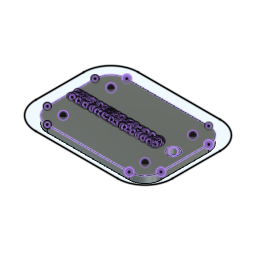
key chain mold v3 (Autodesk Fusion 360 design; units mm, degrees)
Autodesk Fusion 360 part; units mm, degrees
sketch "Sketch1" plane through (0, 0, 0) normal (0, 0, 1) x (1, 0, 0) in component "KEY CHAIN"
  line L0 (0, 0) -> (50, 0)
  line L1 (50, 0) -> (50, 35)
  line L2 (50, 35) -> (0, 35)
  line L3 (0, 35) -> (0, 0)
  dimension "d1" = 50
  dimension "d2" = 35
  constraint horizontal L0
  constraint vertical L1
  constraint horizontal L2
  constraint vertical L3
  constraint coincident L0.start L3.end
  measures "d1" distance of L0.start L0.end
  measures "d2" distance of L0.start L2.end
extrude "Extrude1" add sketch "Sketch1" along normal blind 3 in component "KEY CHAIN"
fillet "Fillet1" radius 7 4 edges at (0, 35, 1.5) (0, 0, 1.5) (50, 0, 1.5) (50, 35, 1.5) in component "KEY CHAIN"
sketch "Sketch2" plane through (0, 0, 3) normal (0, 0, 1) x (-1, 0, 0) in component "KEY CHAIN"
  arc A0 (-50, -28) -> (-43, -35) centre (-43, -28) ccw
  line L0 (-43, -35) -> (-7, -35)
  arc A1 (-7, -35) -> (0, -28) centre (-7, -28) ccw
  line L1 (0, -28) -> (0, -7)
  arc A2 (0, -7) -> (-7, 0) centre (-7, -7) ccw
  line L2 (-7, 0) -> (-43, 0)
  arc A3 (-43, 0) -> (-50, -7) centre (-43, -7) ccw
  line L3 (-50, -7) -> (-50, -28)
  line L4 (-50, -17.5) -> (-45, -17.5) construction
  dimension "d7" = 5
  constraint midpoint L3 L4.start
  constraint perpendicular L3 L4
  measures "d7" distance of L4.start L4.end
hole "Hole1" at (45, 17.5, 3) direction (0, 0, -1) diameter 5 depth 3 tip angle 180 in component "KEY CHAIN"
sketch "Sketch3" plane through (0, 0, 3) normal (0, 0, 1) x (-1, 0, 0) in component "KEY CHAIN"
  circle A0 centre (-45, -17.5) radius 2.5
  arc A1 (-50, -28) -> (-43, -35) centre (-43, -28) ccw
  line L0 (-43, -35) -> (-7, -35)
  arc A2 (-7, -35) -> (0, -28) centre (-7, -28) ccw
  line L1 (0, -28) -> (0, -7)
  arc A3 (0, -7) -> (-7, 0) centre (-7, -7) ccw
  line L2 (-7, 0) -> (-43, 0)
  arc A4 (-43, 0) -> (-50, -7) centre (-43, -7) ccw
  line L3 (-50, -7) -> (-50, -28)
  line L4 (0, 0) -> (-40, 0) construction
  line L5 (-40, 0) -> (-40, -35) construction
  line L6 (-40, -35) -> (0, -35) construction
  line L7 (0, -35) -> (0, 0) construction
  dimension "d11" = 3
  text T0 "PHILLYSNEXT LLC" font "Arial" height 3 bold align centre middle in box 40 x 35 at (0, 0) x (-1, 0) y (0, -1) spacing 1 kerned
  constraint coincident L2
extrude "Extrude2" add sketch "Sketch3" along normal blind 1 text T0 in component "KEY CHAIN"
sketch "Sketch1 (2)" plane through (0, 0, 3) normal (0, 0, 1) x (-1, 0, 0) in component "ONE PART MOLD"
  arc A0 (-50, -28) -> (-43, -35) centre (-43, -28) ccw
  line L0 (-43, -35) -> (-7, -35)
  arc A1 (-7, -35) -> (0, -28) centre (-7, -28) ccw
  line L1 (0, -28) -> (0, -7)
  arc A2 (0, -7) -> (-7, 0) centre (-7, -7) ccw
  line L2 (-7, 0) -> (-43, 0)
  arc A3 (-43, 0) -> (-50, -7) centre (-43, -7) ccw
  line L3 (-50, -7) -> (-50, -28)
  circle A4 centre (-45, -17.5) radius 2.5
  line L4 (-4.1569, -16) -> (-4.1569, -19)
  line L5 (-4.1569, -19) -> (-4.7626, -19)
  line L6 (-4.7626, -19) -> (-4.7626, -17.8192)
  line L7 (-4.7626, -17.8192) -> (-5.9495, -17.8192)
  line L8 (-5.9495, -17.8192) -> (-5.9495, -19)
  line L9 (-5.9495, -19) -> (-6.5553, -19)
  line L10 (-6.5553, -19) -> (-6.5553, -16)
  line L11 (-6.5553, -16) -> (-5.9495, -16)
  line L12 (-5.9495, -16) -> (-5.9495, -17.3117)
  line L13 (-5.9495, -17.3117) -> (-4.7626, -17.3117)
  line L14 (-4.7626, -17.3117) -> (-4.7626, -16)
  line L15 (-4.7626, -16) -> (-4.1569, -16)
  line L16 (-8.3622, -16) -> (-8.3622, -18.9754)
  line L17 (-8.3622, -18.9754) -> (-8.9679, -18.9754)
  line L18 (-8.9679, -18.9754) -> (-8.9679, -16.5055)
  line L19 (-8.9679, -16.5055) -> (-10.4741, -16.5055)
  line L20 (-10.4741, -16.5055) -> (-10.4741, -16)
  line L21 (-10.4741, -16) -> (-8.3622, -16)
  line L22 (-13.869, -16) -> (-13.869, -17.2626)
  line L23 (-13.869, -17.2626) -> (-12.7701, -19)
  line L24 (-12.7701, -19) -> (-13.4802, -19)
  line L25 (-13.4802, -19) -> (-14.1862, -17.8131)
  line L26 (-14.1862, -17.8131) -> (-14.8779, -19)
  line L27 (-14.8779, -19) -> (-15.5757, -19)
  line L28 (-15.5757, -19) -> (-14.4727, -17.2585)
  line L29 (-14.4727, -17.2585) -> (-14.4727, -16)
  line L30 (-14.4727, -16) -> (-13.869, -16)
  line L31 (-38.0532, -17.103) -> (-38.6405, -16.9168)
  spline S0 degree 3 poles (-38.6405, -16.9168) (-38.5921, -16.7668) (-38.5015, -16.4863) (-38.2899, -16.2822) (-38.1913, -16.1872) knots 0 0 0 0 0.04642 0.086856 0.086856 0.086856 0.086856
  spline S1 degree 3 poles (-38.1913, -16.1872) (-38.0756, -16.1178) (-37.8308, -15.9708) (-37.545, -15.9564) (-37.3943, -15.9488) knots 0 0 0 0 0.039867 0.084342 0.084342 0.084342 0.084342
  spline S2 degree 3 poles (-37.3943, -15.9488) (-37.2051, -15.9646) (-36.8336, -15.9956) (-36.5508, -16.238) (-36.412, -16.3571) knots 0 0 0 0 0.055382 0.108818 0.108818 0.108818 0.108818
  spline S3 degree 3 poles (-36.412, -16.3571) (-36.2999, -16.5125) (-36.0603, -16.8446) (-36.0388, -17.255) (-36.0273, -17.4734) knots 0 0 0 0 0.056279 0.120316 0.120316 0.120316 0.120316
  spline S4 degree 3 poles (-36.0273, -17.4734) (-36.0378, -17.7027) (-36.0574, -18.1287) (-36.3014, -18.4763) (-36.4141, -18.6368) knots 0 0 0 0 0.067232 0.124868 0.124868 0.124868 0.124868
  spline S5 degree 3 poles (-36.4141, -18.6368) (-36.5561, -18.7576) (-36.849, -19.0068) (-37.2332, -19.0361) (-37.4311, -19.0512) knots 0 0 0 0 0.054496 0.112371 0.112371 0.112371 0.112371
  spline S6 degree 3 poles (-37.4311, -19.0512) (-37.6033, -19.04) (-37.9339, -19.0187) (-38.1986, -18.8206) (-38.3254, -18.7258) knots 0 0 0 0 0.05054 0.097009 0.097009 0.097009 0.097009
  spline S7 degree 3 poles (-38.3254, -18.7258) (-38.3904, -18.6507) (-38.531, -18.4883) (-38.5969, -18.2834) (-38.6323, -18.1733) knots 0 0 0 0 0.02949 0.063785 0.063785 0.063785 0.063785
  line L32 (-38.6323, -18.1733) -> (-38.0327, -18.03)
  spline S8 degree 3 poles (-38.0327, -18.03) (-38.011, -18.103) (-37.9687, -18.2451) (-37.8624, -18.3482) (-37.8107, -18.3984) knots 0 0 0 0 0.02243 0.043656 0.043656 0.043656 0.043656
  spline S9 degree 3 poles (-37.8107, -18.3984) (-37.7503, -18.4377) (-37.6256, -18.519) (-37.477, -18.5285) (-37.4004, -18.5334) knots 0 0 0 0 0.021266 0.043851 0.043851 0.043851 0.043851
  spline S10 degree 3 poles (-37.4004, -18.5334) (-37.295, -18.524) (-37.0872, -18.5056) (-36.9344, -18.3638) (-36.8591, -18.294) knots 0 0 0 0 0.030797 0.060705 0.060705 0.060705 0.060705
  spline S11 degree 3 poles (-36.8591, -18.294) (-36.7989, -18.1919) (-36.6586, -17.9543) (-36.654, -17.6767) (-36.6514, -17.5184) knots 0 0 0 0 0.035017 0.081505 0.081505 0.081505 0.081505
  spline S12 degree 3 poles (-36.6514, -17.5184) (-36.6532, -17.3518) (-36.6562, -17.0633) (-36.7967, -16.8135) (-36.8561, -16.708) knots 0 0 0 0 0.048972 0.084763 0.084763 0.084763 0.084763
  spline S13 degree 3 poles (-36.8561, -16.708) (-36.9299, -16.6376) (-37.0791, -16.4954) (-37.2844, -16.4762) (-37.3881, -16.4666) knots 0 0 0 0 0.029695 0.059976 0.059976 0.059976 0.059976
  spline S14 degree 3 poles (-37.3881, -16.4666) (-37.4655, -16.4727) (-37.6185, -16.4848) (-37.7423, -16.5753) (-37.8035, -16.6201) knots 0 0 0 0 0.022784 0.04507 0.04507 0.04507 0.04507
  spline S15 degree 3 poles (-37.8035, -16.6201) (-37.8584, -16.6832) (-37.9803, -16.8234) (-38.0273, -17.0038) (-38.0532, -17.103) knots 0 0 0 0 0.024761 0.055018 0.055018 0.055018 0.055018
  line L33 (-21.6985, -16) -> (-21.6985, -19)
  line L34 (-21.6985, -19) -> (-23.9229, -19)
  line L35 (-23.9229, -19) -> (-23.9229, -18.4925)
  line L36 (-23.9229, -18.4925) -> (-22.3042, -18.4925)
  line L37 (-22.3042, -18.4925) -> (-22.3042, -17.8274)
  line L38 (-22.3042, -17.8274) -> (-23.8104, -17.8274)
  line L39 (-23.8104, -17.8274) -> (-23.8104, -17.322)
  line L40 (-23.8104, -17.322) -> (-22.3042, -17.322)
  line L41 (-22.3042, -17.322) -> (-22.3042, -16.5055)
  line L42 (-22.3042, -16.5055) -> (-23.9802, -16.5055)
  line L43 (-23.9802, -16.5055) -> (-23.9802, -16)
  line L44 (-23.9802, -16) -> (-21.6985, -16)
  line L45 (-27.9645, -16) -> (-27.9645, -18.4925)
  line L46 (-27.9645, -18.4925) -> (-27.0744, -18.4925)
  line L47 (-27.0744, -18.4925) -> (-27.0744, -19)
  line L48 (-27.0744, -19) -> (-29.4584, -19)
  line L49 (-29.4584, -19) -> (-29.4584, -18.4925)
  line L50 (-29.4584, -18.4925) -> (-28.5703, -18.4925)
  line L51 (-28.5703, -18.4925) -> (-28.5703, -16)
  line L52 (-28.5703, -16) -> (-27.9645, -16)
  line L53 (-33.59, -16) -> (-33.59, -18.9754)
  line L54 (-33.59, -18.9754) -> (-34.1958, -18.9754)
  line L55 (-34.1958, -18.9754) -> (-34.1958, -16.5055)
  line L56 (-34.1958, -16.5055) -> (-35.7019, -16.5055)
  line L57 (-35.7019, -16.5055) -> (-35.7019, -16)
  line L58 (-35.7019, -16) -> (-33.59, -16)
  line L59 (-31.03, -16) -> (-31.03, -18.9754)
  line L60 (-31.03, -18.9754) -> (-31.6357, -18.9754)
  line L61 (-31.6357, -18.9754) -> (-31.6357, -16.5055)
  line L62 (-31.6357, -16.5055) -> (-33.1419, -16.5055)
  line L63 (-33.1419, -16.5055) -> (-33.1419, -16)
  line L64 (-33.1419, -16) -> (-31.03, -16)
  line L65 (-24.1889, -16) -> (-25.2142, -17.5655)
  line L66 (-25.2142, -17.5655) -> (-24.2851, -19)
  line L67 (-24.2851, -19) -> (-24.9932, -19)
  line L68 (-24.9932, -19) -> (-25.5948, -18.0362)
  line L69 (-25.5948, -18.0362) -> (-26.1842, -19)
  line L70 (-26.1842, -19) -> (-26.8861, -19)
  line L71 (-26.8861, -19) -> (-25.9529, -17.543)
  line L72 (-25.9529, -17.543) -> (-26.9782, -16)
  line L73 (-26.9782, -16) -> (-26.2476, -16)
  line L74 (-26.2476, -16) -> (-25.5825, -17.0375)
  line L75 (-25.5825, -17.0375) -> (-24.9154, -16)
  line L76 (-24.9154, -16) -> (-24.1889, -16)
  line L77 (-18.678, -16) -> (-18.678, -19)
  line L78 (-18.678, -19) -> (-19.2674, -19)
  line L79 (-19.2674, -19) -> (-20.4952, -16.9966)
  line L80 (-20.4952, -16.9966) -> (-20.4952, -19)
  line L81 (-20.4952, -19) -> (-21.058, -19)
  line L82 (-21.058, -19) -> (-21.058, -16)
  line L83 (-21.058, -16) -> (-20.4502, -16)
  line L84 (-20.4502, -16) -> (-19.2408, -17.9563)
  line L85 (-19.2408, -17.9563) -> (-19.2408, -16)
  line L86 (-19.2408, -16) -> (-18.678, -16)
  line L87 (-15.7231, -16.9761) -> (-16.3124, -17.0334)
  spline S16 degree 3 poles (-16.3124, -17.0334) (-16.3318, -16.9438) (-16.3672, -16.7797) (-16.478, -16.6544) (-16.5283, -16.5975) knots 0 0 0 0 0.026965 0.049368 0.049368 0.049368 0.049368
  spline S17 degree 3 poles (-16.5283, -16.5975) (-16.5901, -16.557) (-16.7229, -16.4699) (-16.8821, -16.4624) (-16.9673, -16.4584) knots 0 0 0 0 0.021772 0.046802 0.046802 0.046802 0.046802
  spline S18 degree 3 poles (-16.9673, -16.4584) (-17.0552, -16.4608) (-17.2133, -16.4652) (-17.3483, -16.5462) (-17.4083, -16.5822) knots 0 0 0 0 0.025843 0.046491 0.046491 0.046491 0.046491
  spline S19 degree 3 poles (-17.4083, -16.5822) (-17.4515, -16.6239) (-17.5343, -16.7037) (-17.5494, -16.8174) (-17.5566, -16.8718) knots 0 0 0 0 0.01744 0.033404 0.033404 0.033404 0.033404
  spline S20 degree 3 poles (-17.5566, -16.8718) (-17.5543, -16.9056) (-17.5497, -16.9716) (-17.5124, -17.0262) (-17.4942, -17.0529) knots 0 0 0 0 0.009971 0.019467 0.019467 0.019467 0.019467
  spline S21 degree 3 poles (-17.4942, -17.0529) (-17.4667, -17.0779) (-17.4031, -17.1358) (-17.3222, -17.1658) (-17.2763, -17.1828) knots 0 0 0 0 0.011054 0.025581 0.025581 0.025581 0.025581
  spline S22 degree 3 poles (-17.2763, -17.1828) (-17.2182, -17.2002) (-17.0578, -17.2483) (-16.8951, -17.2883) (-16.7913, -17.3138) knots 0 0 0 0 0.01818 0.050243 0.050243 0.050243 0.050243
  spline S23 degree 3 poles (-16.7913, -17.3138) (-16.6491, -17.3499) (-16.4045, -17.412) (-16.1954, -17.5519) (-16.1078, -17.6105) knots 0 0 0 0 0.043569 0.074988 0.074988 0.074988 0.074988
  spline S24 degree 3 poles (-16.1078, -17.6105) (-16.0272, -17.6969) (-15.8679, -17.8675) (-15.8436, -18.0995) (-15.8315, -18.2142) knots 0 0 0 0 0.03441 0.068023 0.068023 0.068023 0.068023
  spline S25 degree 3 poles (-15.8315, -18.2142) (-15.8371, -18.2897) (-15.8485, -18.4422) (-15.9236, -18.5756) (-15.9615, -18.6429) knots 0 0 0 0 0.022414 0.045289 0.045289 0.045289 0.045289
  spline S26 degree 3 poles (-15.9615, -18.6429) (-16.0107, -18.7059) (-16.1121, -18.8358) (-16.2599, -18.9091) (-16.3359, -18.9468) knots 0 0 0 0 0.023672 0.048778 0.048778 0.048778 0.048778
  spline S27 degree 3 poles (-16.3359, -18.9468) (-16.4251, -18.9772) (-16.6163, -19.0424) (-16.8185, -19.0481) (-16.9263, -19.0512) knots 0 0 0 0 0.028099 0.060257 0.060257 0.060257 0.060257
  spline S28 degree 3 poles (-16.9263, -19.0512) (-17.0962, -19.0462) (-17.4026, -19.0371) (-17.6613, -18.8755) (-17.7766, -18.8035) knots 0 0 0 0 0.049882 0.089973 0.089973 0.089973 0.089973
  spline S29 degree 3 poles (-17.7766, -18.8035) (-17.8605, -18.7124) (-18.0327, -18.5254) (-18.0616, -18.2723) (-18.0764, -18.1426) knots 0 0 0 0 0.036185 0.074274 0.074274 0.074274 0.074274
  line L88 (-18.0764, -18.1426) -> (-17.4707, -18.116)
  spline S30 degree 3 poles (-17.4707, -18.116) (-17.4565, -18.1855) (-17.4307, -18.312) (-17.3433, -18.4061) (-17.3039, -18.4485) knots 0 0 0 0 0.020795 0.037841 0.037841 0.037841 0.037841
  spline S31 degree 3 poles (-17.3039, -18.4485) (-17.2518, -18.4779) (-17.1333, -18.5448) (-16.9967, -18.548) (-16.9202, -18.5498) knots 0 0 0 0 0.017701 0.040226 0.040226 0.040226 0.040226
  spline S32 degree 3 poles (-16.9202, -18.5498) (-16.8399, -18.5473) (-16.6934, -18.5426) (-16.5649, -18.4729) (-16.5068, -18.4413) knots 0 0 0 0 0.023689 0.043263 0.043263 0.043263 0.043263
  spline S33 degree 3 poles (-16.5068, -18.4413) (-16.4788, -18.4163) (-16.423, -18.3664) (-16.4147, -18.2921) (-16.4106, -18.2551) knots 0 0 0 0 0.010872 0.021632 0.021632 0.021632 0.021632
  spline S34 degree 3 poles (-16.4106, -18.2551) (-16.4148, -18.2206) (-16.4234, -18.1495) (-16.4744, -18.099) (-16.5007, -18.073) knots 0 0 0 0 0.010127 0.020858 0.020858 0.020858 0.020858
  spline S35 degree 3 poles (-16.5007, -18.073) (-16.5653, -18.0379) (-16.7399, -17.943) (-16.9346, -17.8997) (-17.0573, -17.8724) knots 0 0 0 0 0.021964 0.059406 0.059406 0.059406 0.059406
  spline S36 degree 3 poles (-17.0573, -17.8724) (-17.1869, -17.8413) (-17.411, -17.7875) (-17.6221, -17.6954) (-17.7111, -17.6565) knots 0 0 0 0 0.039885 0.06897 0.06897 0.06897 0.06897
  spline S37 degree 3 poles (-17.7111, -17.6565) (-17.7776, -17.6164) (-17.9088, -17.5372) (-17.9984, -17.4129) (-18.0426, -17.3516) knots 0 0 0 0 0.023035 0.045457 0.045457 0.045457 0.045457
  spline S38 degree 3 poles (-18.0426, -17.3516) (-18.0775, -17.2809) (-18.1517, -17.1305) (-18.1586, -16.9627) (-18.1623, -16.8738) knots 0 0 0 0 0.023406 0.049744 0.049744 0.049744 0.049744
  spline S39 degree 3 poles (-18.1623, -16.8738) (-18.1562, -16.7889) (-18.1437, -16.6175) (-18.0609, -16.4669) (-18.0191, -16.3909) knots 0 0 0 0 0.025221 0.050905 0.050905 0.050905 0.050905
  spline S40 degree 3 poles (-18.0191, -16.3909) (-17.9657, -16.3204) (-17.8571, -16.177) (-17.6959, -16.0969) (-17.6139, -16.0563) knots 0 0 0 0 0.026152 0.053189 0.053189 0.053189 0.053189
  spline S41 degree 3 poles (-17.6139, -16.0563) (-17.5167, -16.0244) (-17.3048, -15.955) (-17.0818, -15.9497) (-16.9611, -15.9468) knots 0 0 0 0 0.030541 0.066508 0.066508 0.066508 0.066508
  spline S42 degree 3 poles (-16.9611, -15.9468) (-16.7885, -15.953) (-16.4728, -15.9643) (-16.2075, -16.1332) (-16.0873, -16.2098) knots 0 0 0 0 0.050718 0.092726 0.092726 0.092726 0.092726
  spline S43 degree 3 poles (-16.0873, -16.2098) (-15.9954, -16.3122) (-15.7992, -16.531) (-15.7495, -16.8216) (-15.7231, -16.9761) knots 0 0 0 0 0.040457 0.086402 0.086402 0.086402 0.086402
  line L89 (-10.9222, -16) -> (-10.9222, -18.9754)
  line L90 (-10.9222, -18.9754) -> (-11.528, -18.9754)
  line L91 (-11.528, -18.9754) -> (-11.528, -16.5055)
  line L92 (-11.528, -16.5055) -> (-13.0341, -16.5055)
  line L93 (-13.0341, -16.5055) -> (-13.0341, -16)
  line L94 (-13.0341, -16) -> (-10.9222, -16)
  line L95 (-7.163, -16) -> (-7.163, -19)
  line L96 (-7.163, -19) -> (-7.7688, -19)
  line L97 (-7.7688, -19) -> (-7.7688, -16)
  line L98 (-7.7688, -16) -> (-7.163, -16)
  line L99 (-1.3595, -16) -> (-1.3595, -19)
  line L100 (-1.3595, -19) -> (-2.3315, -19)
  spline S44 degree 3 poles (-2.3315, -19) (-2.484, -19.0012) (-2.7254, -19.003) (-2.964, -18.9679) (-3.0518, -18.955) knots 0 0 0 0 0.045648 0.072262 0.072262 0.072262 0.072262
  spline S45 degree 3 poles (-3.0518, -18.955) (-3.1348, -18.9252) (-3.3039, -18.8645) (-3.423, -18.7299) (-3.4836, -18.6613) knots 0 0 0 0 0.025999 0.052974 0.052974 0.052974 0.052974
  spline S46 degree 3 poles (-3.4836, -18.6613) (-3.5343, -18.5772) (-3.6423, -18.3979) (-3.6523, -18.1883) (-3.6576, -18.0771) knots 0 0 0 0 0.029011 0.061813 0.061813 0.061813 0.061813
  spline S47 degree 3 poles (-3.6576, -18.0771) (-3.6546, -17.9911) (-3.6491, -17.83) (-3.5865, -17.6817) (-3.5573, -17.6126) knots 0 0 0 0 0.02555 0.047881 0.047881 0.047881 0.047881
  spline S48 degree 3 poles (-3.5573, -17.6126) (-3.5225, -17.5538) (-3.4551, -17.44) (-3.3523, -17.357) (-3.3025, -17.3168) knots 0 0 0 0 0.020298 0.039313 0.039313 0.039313 0.039313
  spline S49 degree 3 poles (-3.3025, -17.3168) (-3.2518, -17.2843) (-3.1541, -17.2215) (-3.0423, -17.1899) (-2.9884, -17.1746) knots 0 0 0 0 0.017955 0.034651 0.034651 0.034651 0.034651
  spline S50 degree 3 poles (-2.9884, -17.1746) (-2.9, -17.1622) (-2.6917, -17.1328) (-2.4813, -17.1321) (-2.3602, -17.1317) knots 0 0 0 0 0.026747 0.063035 0.063035 0.063035 0.063035
  line L101 (-2.3602, -17.1317) -> (-1.9652, -17.1317)
  line L102 (-1.9652, -17.1317) -> (-1.9652, -16)
  line L103 (-1.9652, -16) -> (-1.3595, -16)
  line L104 (0, -28) -> (0, -7)
  arc A5 (0, -7) -> (-7, 0) centre (-7, -7) ccw
  line L105 (-7, 0) -> (-43, 0)
  arc A6 (-7, -35) -> (0, -28) centre (-7, -28) ccw
  line L106 (-50, -7) -> (-50, -28)
  line L107 (5, -28) -> (5, -7)
  arc A7 (5, -7) -> (-7, 5) centre (-7, -7) ccw
  line L108 (-7, 5) -> (-43, 5)
  arc A8 (-43, 5) -> (-55, -7) centre (-43, -7) ccw
  line L109 (-55, -7) -> (-55, -28)
  arc A9 (-55, -28) -> (-43, -40) centre (-43, -28) ccw
  line L110 (-43, -40) -> (-7, -40)
  arc A10 (-7, -40) -> (5, -28) centre (-7, -28) ccw
  dimension "d14" = 5
component "KEY CHAIN" placed x (1, 0, 0) y (0, 1, 0) z (0, 0, 1) at (0, 0, 0)
component "ONE PART MOLD" placed x (1, 0, 0) y (0, 1, 0) z (0, 0, 1) at (0, 0, 0) in component "KEY CHAIN"
